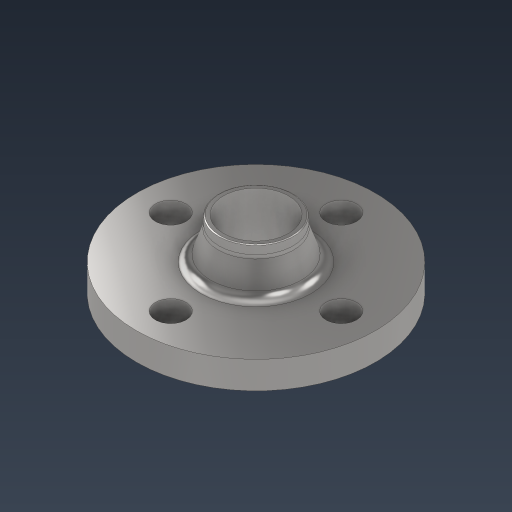
# Autodesk Inventor part: karima
Saved by Autodesk Inventor 2024.3 (Build 283343000, 343)
## iProperties
Created: 2025-10-06
Part Number: karima
Material: Steel, Alloy
Document SubType Name: Modeling
Designer: Agi
Density: 7.73 g/cm^3
Appearance: Semi-Polished
Author: Agi
Autodesk Inventor part; units mm, degrees
ref_plane "YZ Plane" through (0, 0, 0) normal (1, 0, 0) x (0, 1, 0)
ref_plane "XZ Plane" through (0, 0, 0) normal (0, 1, 0) x (-1, 0, 0)
ref_plane "XY Plane" through (0, 0, 0) normal (0, 0, 1) x (1, 0, 0)
sketch "Sketch1" plane through (0, 0, 0) normal (1, 0, 0) x (0, 1, 0)
  line L0 (0, 0) -> (150, 0)
  line L1 (0, 0) -> (0, 39)
  line L2 (0, 39) -> (2, 39)
  line L3 (2, 39) -> (2, 70)
  line L4 (2, 70) -> (18, 70)
  line L5 (18, 70) -> (18, 28)
  line L6 (18, 28) -> (36, 21.75)
  line L7 (36, 21.75) -> (42, 21.75)
  line L8 (42, 21.75) -> (42, 0)
  dimension "d0" = 150
  dimension "d1" = 78
  dimension "d2" = 140
  dimension "d3" = 56
  dimension "d4" = 43.5
  dimension "d5" = 2
  dimension "d6" = 18
  dimension "d7" = 6
  dimension "d8" = 42
  constraints: 18 end point, 5 perpendicular, 1 horizontal, 1 parallel, 1 point on line, 1 vertical
  measures "d0" distance of L0.start L0.end
  measures "d1" diameter of L1.end L0
  measures "d2" diameter of L3.end L0
  measures "d3" diameter of L5.end L0
  measures "d4" diameter of L6.end L0
  measures "d5" distance of L1.end L2.end
  measures "d6" horizontal distance of L1.end L4.end
  measures "d7" distance of L6.end L7.end
  measures "d8" horizontal distance of L1.end L7.end
revolve "Revolution1" add sketch "Sketch1" angle 360 about axis through (0, 0, 0) along (0, 1, 0)
fillet "Fillet1" radius 2 1 edges at (0, 2, -39)
fillet "Fillet2" radius 6 2 edges at (0, 18, -28) (0, 36, -21.75)
chamfer "Chamfer1" distance 0.6 angle 30 1 edges at (0, 42, -21.75) measured on face at (0, 42, -21.25)
sketch "Sketch2" plane through (0, 18, 0) normal (0, 1, 0) x (1, 0, 0)
  point P0 (0, 0)
  point P1 (-50, 0)
  point P2 (0, 50)
  point P3 (50, 0)
  point P4 (0, -50)
hole "Hole1" at (-50, 18, 0) at (0, 18, -50) at (50, 18, 0) at (0, 18, 50) direction (0, -1, 0) diameter 18 end through all
sketch "Sketch4" plane through (0, 42, 0) normal (0, 1, 0) x (1, 0, 0)
  point P0 (0, 0)
  point P1 (0, 0)
  constraints: 1 coincident
hole "Hole2" at (0, 42, 0) direction (0, -1, 0) diameter 38.2 end through all
body "Solid1"
